Autodesk Inventor part; units mm, degrees
(part 2 of 2)
sketch "スケッチ16" plane through (-250, -25, -10) normal (0, -1, 0) x (1, 0, 0)
  line L0 (0, 0) -> (500, 0) projected
  line L1 (51, 0) -> (55, 0)
  line L2 (55, 0) -> (55, -45)
  line L3 (55, -45) -> (51, -45)
  line L4 (51, -45) -> (51, 0)
  line L5 (50, 20) -> (50, 0) projected
  line L6 (298, 20) -> (252.0948, 20) projected
  line L7 (298, 80.5796) -> (252.0948, 20) projected
  line L8 (298, 20) -> (298, 80.5796) projected
  line L9 (302, 78.9446) -> (302, 20) projected
  line L10 (446.2089, 20) -> (302, 78.9446) projected
  line L11 (446.2089, 20) -> (302, 20) projected
  line L12 (252.0948, 99.3431) -> (252.0948, 26.623) projected
  line L13 (294.1682, 82.1459) -> (252.0948, 99.3431) projected
  line L14 (252.0948, 26.623) -> (294.1682, 82.1459) projected
  line L15 (17.9849, 10) -> (4, 6.0772) projected
  line L16 (4, 6.0772) -> (4, 13.9228) projected
  line L17 (4, 13.9228) -> (17.9849, 10) projected
  line L18 (109.9232, 4) -> (125, 7.9331) projected
  line L19 (125, 7.9331) -> (140.0768, 4) projected
  line L20 (140.0768, 4) -> (109.9232, 4) projected
  line L21 (209.9232, 4) -> (225, 7.9331) projected
  line L22 (225, 7.9331) -> (240.0768, 4) projected
  line L23 (240.0768, 4) -> (209.9232, 4) projected
  line L24 (325, 12.0669) -> (309.9232, 16) projected
  line L25 (309.9232, 16) -> (340.0768, 16) projected
  line L26 (340.0768, 16) -> (325, 12.0669) projected
  line L27 (425, 12.0669) -> (409.9232, 16) projected
  line L28 (409.9232, 16) -> (440.0768, 16) projected
  line L29 (440.0768, 16) -> (425, 12.0669) projected
  line L30 (496, 13.9228) -> (496, 6.0772) projected
  line L31 (496, 6.0772) -> (482.0151, 10) projected
  line L32 (482.0151, 10) -> (496, 13.9228) projected
  line L33 (398, 6.0669) -> (382.9232, 10) projected
  line L34 (382.9232, 10) -> (398, 13.9331) projected
  line L35 (398, 13.9331) -> (398, 6.0669) projected
  line L36 (298, 6.0669) -> (282.9232, 10) projected
  line L37 (282.9232, 10) -> (298, 13.9331) projected
  line L38 (298, 13.9331) -> (298, 6.0669) projected
  line L39 (182.9232, 10) -> (198, 13.9331) projected
  line L40 (198, 13.9331) -> (198, 6.0669) projected
  line L41 (198, 6.0669) -> (182.9232, 10) projected
  line L42 (90.0768, 16) -> (75, 12.0669) projected
  line L43 (75, 12.0669) -> (60.1439, 15.9424) projected
  line L44 (60.1439, 15.9424) -> (60, 16) projected
  line L45 (60, 16) -> (90.0768, 16) projected
  line L46 (39.375, 16) -> (25.3901, 12.0772) projected
  line L47 (25.3901, 12.0772) -> (11.4052, 16) projected
  line L48 (11.4052, 16) -> (39.375, 16) projected
  line L49 (132.9232, 10) -> (148, 13.9331) projected
  line L50 (148, 13.9331) -> (148, 6.0669) projected
  line L51 (148, 6.0669) -> (132.9232, 10) projected
  line L52 (232.9232, 10) -> (248, 13.9331) projected
  line L53 (248, 13.9331) -> (248, 6.0669) projected
  line L54 (248, 6.0669) -> (232.9232, 10) projected
  line L55 (348, 6.0669) -> (332.9232, 10) projected
  line L56 (332.9232, 10) -> (348, 13.9331) projected
  line L57 (348, 13.9331) -> (348, 6.0669) projected
  line L58 (448, 6.0669) -> (432.9232, 10) projected
  line L59 (432.9232, 10) -> (448, 13.9331) projected
  line L60 (448, 13.9331) -> (448, 6.0669) projected
  line L61 (474.6099, 12.0772) -> (460.625, 16) projected
  line L62 (460.625, 16) -> (488.5948, 16) projected
  line L63 (488.5948, 16) -> (474.6099, 12.0772) projected
  line L64 (375, 12.0669) -> (359.9232, 16) projected
  line L65 (359.9232, 16) -> (390.0768, 16) projected
  line L66 (390.0768, 16) -> (375, 12.0669) projected
  line L67 (275, 12.0669) -> (259.9232, 16) projected
  line L68 (259.9232, 16) -> (290.0768, 16) projected
  line L69 (290.0768, 16) -> (275, 12.0669) projected
  line L70 (159.9232, 4) -> (175, 7.9331) projected
  line L71 (175, 7.9331) -> (190.0768, 4) projected
  line L72 (190.0768, 4) -> (159.9232, 4) projected
  line L73 (67.0768, 10) -> (52, 6.0669) projected
  line L74 (52, 6.0669) -> (52, 13.9331) projected
  line L75 (52, 13.9331) -> (67.0768, 10) projected
  line L76 (25.3901, 7.9228) -> (40.5948, 3.6579) projected
  line L77 (40.5948, 3.6579) -> (10.1855, 3.6579) projected
  line L78 (10.1855, 3.6579) -> (25.3901, 7.9228) projected
  line L79 (102, 6.0669) -> (102, 13.9331) projected
  line L80 (102, 13.9331) -> (117.0768, 10) projected
  line L81 (117.0768, 10) -> (102, 6.0669) projected
  line L82 (202, 6.0669) -> (202, 13.9331) projected
  line L83 (202, 13.9331) -> (217.0768, 10) projected
  line L84 (217.0768, 10) -> (202, 6.0669) projected
  line L85 (317.0768, 10) -> (302, 6.0669) projected
  line L86 (302, 6.0669) -> (302, 13.9331) projected
  line L87 (302, 13.9331) -> (317.0768, 10) projected
  line L88 (417.0768, 10) -> (402, 6.0669) projected
  line L89 (402, 6.0669) -> (402, 13.9331) projected
  line L90 (402, 13.9331) -> (417.0768, 10) projected
  line L91 (390.0768, 4) -> (359.9232, 4) projected
  line L92 (359.9232, 4) -> (375, 7.9331) projected
  line L93 (375, 7.9331) -> (390.0768, 4) projected
  line L94 (290.0768, 4) -> (259.9232, 4) projected
  line L95 (259.9232, 4) -> (275, 7.9331) projected
  line L96 (275, 7.9331) -> (290.0768, 4) projected
  line L97 (175, 12.0669) -> (159.9232, 16) projected
  line L98 (159.9232, 16) -> (190.0768, 16) projected
  line L99 (190.0768, 16) -> (175, 12.0669) projected
  line L100 (75, 7.9331) -> (89.8561, 4.0576) projected
  line L101 (89.8561, 4.0576) -> (90, 4) projected
  line L102 (90, 4) -> (59.9232, 4) projected
  line L103 (59.9232, 4) -> (75, 7.9331) projected
  line L104 (48, 14.2649) -> (48, 5.7351) projected
  line L105 (48, 5.7351) -> (32.7954, 10) projected
  line L106 (32.7954, 10) -> (48, 14.2649) projected
  line L107 (125, 12.0669) -> (109.9232, 16) projected
  line L108 (109.9232, 16) -> (140.0768, 16) projected
  line L109 (140.0768, 16) -> (125, 12.0669) projected
  line L110 (225, 12.0669) -> (209.9232, 16) projected
  line L111 (209.9232, 16) -> (240.0768, 16) projected
  line L112 (240.0768, 16) -> (225, 12.0669) projected
  line L113 (340.0768, 4) -> (309.9232, 4) projected
  line L114 (309.9232, 4) -> (325, 7.9331) projected
  line L115 (325, 7.9331) -> (340.0768, 4) projected
  line L116 (440.0768, 4) -> (409.9232, 4) projected
  line L117 (409.9232, 4) -> (425, 7.9331) projected
  line L118 (425, 7.9331) -> (440.0768, 4) projected
  line L119 (467.2046, 10) -> (452, 5.7351) projected
  line L120 (452, 5.7351) -> (452, 14.2649) projected
  line L121 (452, 14.2649) -> (467.2046, 10) projected
  line L122 (367.0768, 10) -> (352, 6.0669) projected
  line L123 (352, 6.0669) -> (352, 13.9331) projected
  line L124 (352, 13.9331) -> (367.0768, 10) projected
  line L125 (267.0768, 10) -> (252, 6.0669) projected
  line L126 (252, 6.0669) -> (252, 13.9331) projected
  line L127 (252, 13.9331) -> (267.0768, 10) projected
  line L128 (152, 6.0669) -> (152, 13.9331) projected
  line L129 (152, 13.9331) -> (167.0768, 10) projected
  line L130 (167.0768, 10) -> (152, 6.0669) projected
  line L131 (98, 13.9331) -> (98, 6.0669) projected
  line L132 (98, 6.0669) -> (82.9232, 10) projected
  line L133 (82.9232, 10) -> (98, 13.9331) projected
  line L134 (459.4052, 3.6579) -> (474.6099, 7.9228) projected
  line L135 (474.6099, 7.9228) -> (489.8145, 3.6579) projected
  line L136 (489.8145, 3.6579) -> (459.4052, 3.6579) projected
  line L137 (198, 78.9446) -> (198, 20) projected
  line L138 (198, 20) -> (53.7911, 20) projected
  line L139 (53.7911, 20) -> (198, 78.9446) projected
  line L140 (250, 104.5206) -> (456.7809, 20) projected
  line L141 (250, 104.5206) -> (43.2191, 20) projected
  line L142 (43.2191, 20) -> (0, 20) projected
  line L143 (0, 0) -> (0, 20) projected
  line L144 (0, 0) -> (500, 0) projected
  line L145 (500, 20) -> (500, 0) projected
  line L146 (500, 20) -> (456.7809, 20) projected
  line L147 (247.9052, 26.623) -> (205.8318, 82.1459) projected
  line L148 (205.8318, 82.1459) -> (247.9052, 99.3431) projected
  line L149 (247.9052, 99.3431) -> (247.9052, 26.623) projected
  line L150 (247.9052, 20) -> (202, 20) projected
  line L151 (202, 20) -> (202, 80.5796) projected
  line L152 (202, 80.5796) -> (247.9052, 20) projected
  line L153 (102, 4) -> (102, 0) projected
  line L154 (55, -45) -> (250, 0)
  line L155 (98, 0) -> (77.9662, 0) projected
  line L156 (232.2111, 0) -> (55, -40.8949)
  point P0 (250, 10)
  dimension "d148" = 4
  dimension "d149" = 45
  dimension "d150" = 1
  dimension "d151" = 4
  constraints: 12 end point, 3 parallel, 3 point on line, 2 midpoint, 1 horizontal, 1 perpendicular
  measures "d148" distance of L2.end L3.end
  measures "d149" distance of L1.end L2.end
  measures "d150" distance between parallel lines of L4 L5
  measures "d151" distance between parallel lines of L154 L156
sketch "スケッチ17" plane through (-250, 25, -10) normal (0, 1, 0) x (1, 0, 0)
  point P0 (250, -10)
